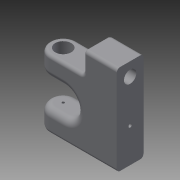
# Autodesk Inventor part: lickometer
Saved by Autodesk Inventor 2015 (Build 190159000, 159)
## iProperties
Created: 2015-08-17
Part Number: lickometer
Material: Generic
Document SubType Name: Modeling
Designer: Lapis
Density: 1 g/cm^3
Appearance: Default
Author: Lapis
Autodesk Inventor part; units mm, degrees
ref_plane "YZ Plane" through (0, 0, 0) normal (1, 0, 0) x (0, 1, 0)
ref_plane "XZ Plane" through (0, 0, 0) normal (0, 1, 0) x (-1, 0, 0)
ref_plane "XY Plane" through (0, 0, 0) normal (0, 0, 1) x (1, 0, 0)
sketch "Sketch1" plane through (0, 0, 0) normal (0, 0, 1) x (1, 0, 0)
  line L0 (0, 4) -> (20, 4)
  line L1 (20, 4) -> (20, -4)
  line L2 (20, -4) -> (0, -4)
  arc A0 (0, 4) -> (0, -4) centre (0, 0) ccw
  dimension "d0" = 20
  dimension "d1" = 8
  constraints: 6 end point, 2 perpendicular, 2 point on circle, 2 tangent, 1 centre point, 1 coincident, 1 horizontal
  measures "d0" distance of L0.start L0.end
  measures "d1" distance of L0.end L1.end
extrude "Extrusion1" add sketch "Sketch1" along normal mid plane 20.4
sketch "Sketch2" plane through (0, 0, 0) normal (0, 1, 0) x (-1, 0, 0)
  line L0 (4, -10.2) -> (4, 10.2) projected
  line L1 (4, 4) -> (-4, 4)
  line L2 (4, -4) -> (-4, -4)
  arc A0 (-4, 4) -> (-4, -4) centre (-4, 0) ccw
  point P0 (0, 0)
  dimension "d4" = 8
  dimension "d5" = 8
  constraints: 4 end point, 2 point on circle, 2 point on line, 2 tangent, 1 centre point, 1 horizontal, 1 horizontal alignment, 1 perpendicular
  measures "d4" distance between parallel lines of L2 L1
  measures "d5" distance of L2.start L2.end
extrude "Extrusion2" cut sketch "Sketch2" along normal through all both and the other way through all
sketch "Sketch3" plane through (0, 0, -10.2) normal (0, 0, -1) x (-1, 0, 0)
  circle A0 centre (0, 0) radius 2.4
  dimension "d8" = 4.8
  constraints: 1 centre point, 1 coincident
  measures "d8" diameter of A0
extrude "Extrusion3" cut sketch "Sketch3" against normal blind 4.1
sketch "Sketch4" plane through (0, 0, 0) normal (1, 0, 0) x (0, 1, 0)
  line L0 (-4, -4) -> (4, -4) projected
  line L1 (4, -4) -> (4, -10.2) projected
  line L2 (4, -10.2) -> (2.4, -10.2) projected
  line L3 (2.4, -10.2) -> (2.4, -6.1) projected
  line L4 (2.4, -6.1) -> (-2.4, -6.1) projected
  line L5 (-2.4, -6.1) -> (-2.4, -10.2) projected
  line L6 (-2.4, -10.2) -> (-4, -10.2) projected
  line L7 (-4, -10.2) -> (-4, -4) projected
  line L8 (4, 4) -> (-4, 4) projected
  line L9 (-4, 4) -> (-4, 10.2) projected
  line L10 (-4, 10.2) -> (4, 10.2) projected
  line L11 (4, 10.2) -> (4, 4) projected
  arc A0 (0, -4.4) -> (-2.4, -6.1) centre (0, -6.9441) ccw
  line L12 (0, -4.4) -> (0, -6.1)
  point P0 (0, 0)
  dimension "d11" = 1.7
  constraints: 2 end point, 2 point on circle, 2 vertical alignment, 1 centre point, 1 midpoint
  measures "d11" distance from line of L4 L12.start
revolve "Revolution1" cut sketch "Sketch4" angle 360 about axis through (0, 0, -4.4) along (0, 0, -1) contours A0 L12 L4
mirror "Mirror1" about plane through (0, 0, 0) normal (0, 0, 1) of "Revolution1", "Extrusion3"
sketch "Sketch5" plane through (0, 0, -10.2) normal (0, 0, -1) x (-1, 0, 0)
  point P0 (0, 0)
  point P1 (0, 0)
  constraints: 1 coincident
hole "Hole1" at (0, 0, -10.2) direction (0, 0, 1) diameter 0.75 end through all
sketch "Sketch6" plane through (20, -4, 10.2) normal (1, 0, 0) x (0, 0, -1)
  point P0 (10.2, 4)
  point P1 (10.2, 4)
  constraints: 1 coincident
hole "Hole2" at (20, 0, 0) direction (-1, 0, 0) diameter 1 end through all
sketch "Sketch9" plane through (20, -4, 10.2) normal (1, 0, 0) x (0, 0, -1)
  line L0 (-6.5, 8) -> (-6.5, 0)
  line L1 (-6.5, 0) -> (6.2, 0)
  line L2 (6.2, 0) -> (6.2, 8)
  line L3 (6.2, 8) -> (-6.5, 8)
  point P0 (10.2, 4)
  point P1 (-6.5, 4)
  point P2 (6.2, 4)
  dimension "d34" = 8
  dimension "d35" = 12.7
  dimension "d36" = 4
  constraints: 8 end point, 3 perpendicular, 2 horizontal alignment, 2 midpoint, 1 vertical
  measures "d34" distance of L0.start L0.end
  measures "d35" distance of L0.end L1.end
  measures "d36" distance from line of point (10.2, 4) L2
extrude "Extrusion6" add sketch "Sketch9" against normal blind 10
sketch "Sketch10" plane through (20, -4, -10.2) normal (1, 0, 0) x (0, 0, -1)
  point P0 (-10.2, 4)
  point P1 (-22.9, 4)
  dimension "d39" = 12.7
  constraints: 1 horizontal alignment
  measures "d39" distance of point (-10.2, 4) point (-22.9, 4)
hole "Hole3" at (20, 0, 12.7) direction (-1, 0, 0) diameter 3.7 end through all
fillet "Fillet1" radius 1 12 edges at (10, 4, -10.2) (10, -4, -10.2) (-4, 0, -10.2) (-4, 0, 10.2) (5, -4, 10.2) (5, 4, 10.2) (10, 4, 13.45) (10, -4, 13.45) (10, 0, 10.2) (15, 4, 16.7) (15, -4, 16.7) (10, 0, 16.7)
fillet "Fillet1" radius 2 8 edges at (2, 4, -4) (8, 4, 0) (2, 4, 4) (-4, 0, 4) (2, -4, 4) (8, -4, 0) (2, -4, -4) (-4, 0, -4)
body "Solid1"
